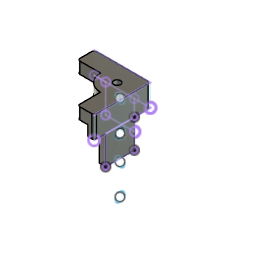
idler-profile connector 2 (Autodesk Fusion 360 design; units mm, degrees)
Autodesk Fusion 360 part; units mm, degrees
sketch "Sketch1" plane through (0, 0, 40) normal (0, 0, 1) x (-1, 0, 0)
  line L0 (-23.5, -15) -> (-29, -15)
  line L1 (-29, -15) -> (-29, -29)
  line L2 (-29, -29) -> (-15, -29)
  line L3 (-15, -29) -> (-15, -23.5)
  line L4 (-15, -23.5) -> (10, -23.5)
  line L5 (10, -23.5) -> (10, -29)
  line L6 (10, -29) -> (20, -29)
  line L7 (20, -29) -> (20, -20)
  line L8 (20, -20) -> (20, -14.5)
  line L9 (20, -14.5) -> (0, -14.5)
  arc A0 (0, -14.5) -> (-14.5, 0) centre (-14.5, -14.5) ccw
  line L10 (-14.5, 0) -> (-14.5, 20)
  line L11 (-14.5, 20) -> (-29, 20)
  line L12 (-29, 20) -> (-29, 10)
  line L13 (-29, 10) -> (-23.5, 10)
  line L14 (-23.5, 10) -> (-23.5, -15)
  circle A1 centre (-14.5, -14.5) radius 1.5
  line L15 (-29, 20) -> (-29, -29)
  line L16 (-29, -29) -> (20, -29)
  line L17 (-15, -23.5) -> (20, -23.5)
  line L18 (-15, -23.5) -> (-29, -23.5527)
  line L19 (-23.5, -15) -> (-23.5726, -29)
  line L20 (-23.5, 10) -> (-23.5, 20)
  constraint coincident L11.end L12.start
  constraint coincident L1.end L2.start
  constraint coincident L6.end L7.start
  constraint coincident L3.end L4.start
  constraint coincident L7 L17.end
  constraint perpendicular L7 L17
  constraint coincident L15 L18.end
  constraint coincident L0.start L14.end
  constraint coincident L16 L19.end
  constraint coincident L13.end L14.start
  constraint coincident L11 L20.end
  constraint perpendicular L11 L20
extrude "Extrude1" add sketch "Sketch1" along normal blind 9 contours L0 L1 L15 L18 L19 | L0 L13 L14 L15 | L11 L12 L13 L15 L20 | L1 L2 L15 L16 L18 L19 | L2 L3 L16 L18 L19 | L3 L4 L5 L16 L17 | L5 L6 L7 L16 L17
extrude "Extrude2" add sketch "Sketch1" against normal blind 25 contours L0 L13 L14 L15 | L3 L4 L5 L16 L17
extrude "Extrude8" add sketch "Sketch1" along normal blind 10 from surface at 9
sketch "Sketch3" plane through (29, 0, 0) normal (1, 0, 0) x (0, 1, 0)
  line L0 (-20, 40) -> (-10, 40)
  line L1 (29, 40) -> (29, 59)
  line L2 (-20, 59) -> (-20, 40)
  circle A0 centre (2.5, 34) radius 2.1
  circle A1 centre (2.5, 34) radius 4
  circle A2 centre (2.5, -14) radius 2.1
  circle A3 centre (2.5, -14) radius 4
  line L3 (-20, 40) -> (29, 40)
  line L4 (-10, 40) -> (-10, 15)
  line L5 (-10, 15) -> (15, 15)
  line L6 (15, 15) -> (15, 40)
  line L7 (15, 40) -> (29, 40)
  line L8 (29, 59) -> (-20, 59)
  dimension "d5" = 4.2
  dimension "d6" = 8
  dimension "d7" = 4.2
  dimension "d8" = 8
  dimension "d10" = 6
  constraint concentric A0 A1
  constraint concentric A2 A3
  measures "d5" diameter of A0
  measures "d6" diameter of A1
  measures "d7" diameter of A2
  measures "d8" diameter of A3
  measures "d10" distance of A0.centre L3
extrude "Extrude3" cut sketch "Sketch3" against normal blind 5.5 contours A0 | A2
extrude "Extrude4" cut sketch "Sketch3" against normal blind 4 contours A1 | A3
sketch "Sketch4" plane through (0, 29, 0) normal (0, 1, 0) x (-1, 0, 0)
  line L0 (-29, 40) -> (-15, 40)
  line L1 (20, 40) -> (20, 59)
  line L2 (-29, 59) -> (-29, 40)
  circle A0 centre (-2.5, 34) radius 2.1
  circle A1 centre (-2.5, 34) radius 4
  circle A2 centre (-2.5, -14) radius 2.1
  circle A3 centre (-2.5, -14) radius 4
  line L3 (-29, 40) -> (20, 40)
  line L4 (-15, 40) -> (-15, 15)
  line L5 (-15, 15) -> (10, 15)
  line L6 (10, 15) -> (10, 40)
  line L7 (10, 40) -> (20, 40)
  line L8 (20, 59) -> (-29, 59)
  dimension "d15" = 4.2
  dimension "d16" = 8
  dimension "d17" = 4.2
  dimension "d18" = 8
  dimension "d20" = 6
  constraint concentric A0 A1
  constraint concentric A2 A3
  measures "d15" diameter of A0
  measures "d16" diameter of A1
  measures "d17" diameter of A2
  measures "d18" diameter of A3
  measures "d20" distance of A0.centre L3
extrude "Extrude5" cut sketch "Sketch4" against normal blind 5.5 contours A0 | A2
extrude "Extrude6" cut sketch "Sketch4" against normal blind 4 contours A1 | A3
sketch "Sketch6" plane through (0, 0, 59) normal (0, 0, 1) x (-1, 0, 0)
  circle A0 centre (-14.5, -14.5) radius 1.5
  line L0 (-29, -29) -> (20, -29)
  line L1 (20, -29) -> (20, -20)
  line L2 (20, -20) -> (20, -14.5)
  line L3 (20, -14.5) -> (0, -14.5)
  arc A1 (0, -14.5) -> (-14.5, 0) centre (-14.5, -14.5) ccw
  line L4 (-14.5, 0) -> (-14.5, 20)
  line L5 (-14.5, 20) -> (-29, 20)
  line L6 (-29, 20) -> (-29, -29)
  circle A2 centre (-14.5, -14.5) radius 1.5
  circle A3 centre (-14.5, -14.5) radius 3
  dimension "d34" = 6
  constraint concentric A0 A2
  constraint concentric A0 A3
  measures "d34" diameter of A3
extrude "Extrude7" cut sketch "Sketch6" against normal blind 4 contours A3
move_face "OffsetFaces1" offset -0.2 1 faces at (13.0075, 14.6494, 51)
fillet "Fillet1" radius 2 5 edges at (-20, 14.5, 54) (14.5, -20, 54) (-20, 29, 49.5) (29, 29, 49.5) (29, -20, 49.5)
